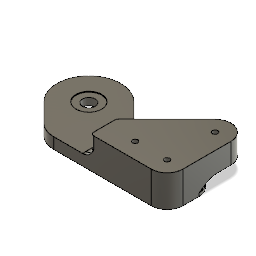
grt_knee_inner_20190218 (Autodesk Fusion 360 archive; units mm, degrees)
design "grt_knee_inner"
Autodesk Fusion 360 part; units mm, degrees
sketch "Skizze1" plane through (0, 0, 0) normal (0, 1, 0) x (1, 0, 0)
  circle A0 centre (0, 0) radius 4
  line L0 (7.9289, -30) -> (69, -30)
  line L1 (79, -20) -> (79, -10)
  circle A1 centre (0, 0) radius 20
  line L2 (-2.6777, -25.6066) -> (-14.1421, -14.1421)
  line L3 (23.8909, 4.3934) -> (14.1421, 14.1421)
  line L4 (34.4975, 0) -> (69, 0)
  arc A2 (23.8909, 4.3934) -> (34.4975, 0) centre (34.4975, 15) ccw
  arc A3 (-2.6777, -25.6066) -> (7.9289, -30) centre (7.9289, -15) ccw
  arc A4 (79, -10) -> (69, 0) centre (69, -10) ccw
  arc A5 (69, -30) -> (79, -20) centre (69, -20) ccw
  dimension "d4" = 8
  dimension "d46" = 30
  dimension "d83" = 40
  dimension "d84" = 135
  dimension "d85" = 15
  dimension "d86" = 15
  dimension "d87" = 10
  dimension "d103" = 79
  dimension "d107" = 10
  dimension "d108" = 30
  dimension "d117" = 0
  dimension "d118" = 0
  dimension "d119" = 0
  dimension "d120" = 0
  dimension "d152" = 0
  dimension "d153" = 0
  dimension "d154" = 0
  dimension "d155" = 0
  measures "d4" diameter of A0
  measures "d46" distance of L0
  measures "d83" diameter of A1
  measures "d84" angle of L3 L4
  measures "d85" radius of A2
  measures "d86" radius of A3
  measures "d87" radius of A4
  measures "d103" distance of L1 A0.centre
  measures "d107" radius of A5
  measures "d108" distance of L0 L4
sketch "Skizze3" plane through (0, 0, 0) normal (0, 1, 0) x (1, 0, 0)
  line L0 (69, -30) -> (33, -30)
  line L1 (31, -28) -> (31, -14.6863)
  line L2 (79, -20) -> (79, 10)
  arc A0 (69, -30) -> (79, -20) centre (69, -20) ccw
  line L3 (31.5858, -13.2721) -> (61.9289, 17.0711)
  arc A1 (79, 10) -> (61.9289, 17.0711) centre (69, 10) ccw
  arc A2 (31, -28) -> (33, -30) centre (33, -28) ccw
  arc A3 (31.5858, -13.2721) -> (31, -14.6863) centre (33, -14.6863) ccw
  dimension "d101" = 25
  dimension "d105" = 10
  dimension "d125" = 30
  dimension "d126" = 79
  dimension "d127" = 10
  dimension "d130" = 135
  dimension "d131" = 2
  dimension "d132" = 2
  dimension "d134" = 31
  dimension "d147" = 30
  measures "d101" distance of origin
  measures "d105" radius of A0
  measures "d126" distance of origin L2
  measures "d127" radius of A1
  measures "d130" angle of L1 L3
  measures "d131" radius of A2
  measures "d132" radius of A3
  measures "d134" distance of origin L1
extrude "Extrusion15" add sketch "Skizze1" against normal blind 7
extrude "Extrusion16" add sketch "Skizze3" along normal blind 13
fillet "Abrundung3" radius 5 4 edges at (38.2218, 0, 6.636) (31.1522, 0, 13.9209) (31, 0, 21.3431) (31.5858, 0, 29.4142)
fillet "Abrundung4" radius 5 2 edges at (76.0711, 0, 2.9289) (56.9289, 0, 0)
sketch "Skizze6" plane through (0, 13, 0) normal (0, 1, 0) x (1, 0, 0)
  arc A0 (69, -30) -> (79, -20) centre (69, -20) ccw
  line L0 (33, -30) -> (69, -30)
  arc A1 (31, -28) -> (33, -30) centre (33, -28) ccw
  line L1 (31, -14.6863) -> (31, -28)
  arc A2 (31.5858, -13.2721) -> (31, -14.6863) centre (33, -14.6863) ccw
  line L2 (61.9289, 17.0711) -> (31.5858, -13.2721)
  arc A3 (79, 10) -> (61.9289, 17.0711) centre (69, 10) ccw
  line L3 (79, -20) -> (79, 10)
  circle A4 centre (69, -20) radius 1.65
  circle A5 centre (69, 10) radius 1.65
  circle A6 centre (49, -20) radius 1.65
  line L4 (7.9289, -30) -> (69, -30)
  line L5 (79, -10) -> (79, -20)
  dimension "d141" = 3.3
  dimension "d143" = 30
  dimension "d144" = 20
  dimension "d171" = 10
  measures "d141" diameter of A4
  measures "d143" distance of L5
extrude "Extrusion20" cut sketch "Skizze6" against normal blind 20 contours A4 | A5 | A6
sketch "Sketch9" plane through (0, 0, 0) normal (0, 1, 0) x (-1, 0, 0)
  line L0 (-28.0503, 9.7365) -> (-37.7868, 0)
  line L1 (-37.7868, 0) -> (-34.4975, 0)
  arc A0 (-23.8909, -4.3934) -> (-34.4975, 0) centre (-34.4975, -15) ccw
  line L2 (-23.8909, -4.3934) -> (-14.1421, -14.1421)
  arc A1 (-14.1421, -14.1421) -> (14.1421, 14.1421) centre (0, 0) ccw
  line L3 (14.1421, 14.1421) -> (2.6777, 25.6066)
  arc A2 (2.6777, 25.6066) -> (-7.9289, 30) centre (-7.9289, 15) ccw
  line L4 (-7.9289, 30) -> (-26.2918, 30)
  arc A3 (-26, 28) -> (-26.2918, 30) centre (-33, 28) ccw
  line L5 (-26, 28) -> (-26, 14.6863)
  arc A4 (-28.0503, 9.7365) -> (-26, 14.6863) centre (-33, 14.6863) ccw
  circle A5 centre (0, 0) radius 4
  circle A6 centre (0, 0) radius 8.05
  dimension "d174" = 16.1
  measures "d174" diameter of A6
extrude "Extrude21" cut sketch "Sketch9" against normal blind 0.5 contours A6
sketch "Sketch10" plane through (0, -7, 0) normal (0, -1, 0) x (1, 0, 0)
  circle A0 centre (69, 20) radius 1.65
  circle A1 centre (49, 20) radius 1.65
  circle A2 centre (0, 0) radius 4
  arc A3 (7.9289, 30) -> (-2.6777, 25.6066) centre (7.9289, 15) ccw
  line L0 (-2.6777, 25.6066) -> (-14.1421, 14.1421)
  arc A4 (-14.1421, 14.1421) -> (14.1421, -14.1421) centre (0, 0) ccw
  line L1 (14.1421, -14.1421) -> (23.8909, -4.3934)
  arc A5 (34.4975, 0) -> (23.8909, -4.3934) centre (34.4975, -15) ccw
  line L2 (34.4975, 0) -> (69, 0)
  arc A6 (69, 0) -> (79, 10) centre (69, 10) ccw
  line L3 (79, 10) -> (79, 20)
  arc A7 (79, 20) -> (69, 30) centre (69, 20) ccw
  line L4 (69, 30) -> (7.9289, 30)
  circle A8 centre (0, 0) radius 8.05
  dimension "d177" = 16.1
  measures "d177" diameter of A8
extrude "Extrude22" cut sketch "Sketch10" against normal blind 2 contours A8
